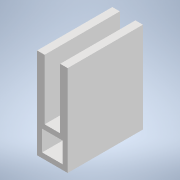
# Autodesk Inventor part: fuselage_tail_interface_front
Saved by Autodesk Inventor 2021 (Build 250183000, 183)
## iProperties
Created: 2020-12-06
Part Number: fuselage_tail_interface_front
Material: Generic
Document SubType Name: Modeling
Designer: victo
Density: 1 g/cm^3
Appearance: Default
Mass: 0.846 g
Surface Area: 14.448 cm^2
Volume: 0.846 cm^3
Author: victo
Autodesk Inventor part; units mm, degrees
ref_plane "YZ Plane" through (0, 0, 0) normal (1, 0, 0) x (0, 1, 0)
ref_plane "XZ Plane" through (0, 0, 0) normal (0, 1, 0) x (-1, 0, 0)
ref_plane "XY Plane" through (0, 0, 0) normal (0, 0, 1) x (1, 0, 0)
sketch "Sketch1" plane through (0, 0, 0) normal (0, 0, 1) x (1, 0, 0)
  line L0 (-3.05, 3.05) -> (3.05, 3.05)
  line L1 (3.05, 3.05) -> (3.05, -3.05)
  line L2 (3.05, -3.05) -> (-3.05, -3.05)
  line L3 (-3.05, -3.05) -> (-3.05, 3.05)
  line L4 (-3.05, 3.05) -> (3.05, -3.05) construction
  line L5 (3.05, 3.05) -> (-3.05, -3.05) construction
  line L6 (-2.05, 2.05) -> (2.05, 2.05)
  line L7 (2.05, 2.05) -> (2.05, -2.05)
  line L8 (2.05, -2.05) -> (-2.05, -2.05)
  line L9 (-2.05, -2.05) -> (-2.05, 2.05)
  line L10 (-2.05, 2.05) -> (2.05, -2.05) construction
  line L11 (2.05, 2.05) -> (-2.05, -2.05) construction
  line L12 (-3.05, 3.05) -> (-1.55, 3.05)
  line L13 (-1.55, 3.05) -> (-1.55, 15.05)
  line L14 (-1.55, 15.05) -> (-3.05, 15.05)
  line L15 (-3.05, 15.05) -> (-3.05, 3.05)
  line L16 (3.05, 3.05) -> (1.55, 3.05)
  line L17 (1.55, 3.05) -> (1.55, 15.05)
  line L18 (1.55, 15.05) -> (3.05, 15.05)
  line L19 (3.05, 15.05) -> (3.05, 3.05)
  point P0 (0, 0)
  point P1 (1.55, 3.05)
  point P2 (-1.55, 3.05)
  dimension "d0" = 6.1
  dimension "d1" = 6.1
  dimension "d2" = 4.1
  dimension "d3" = 4.1
  dimension "d4" = 12
  dimension "d5" = 12
  dimension "d6" = 1.5
  dimension "d7" = 1.5
  constraints: 40 end point, 8 parallel, 4 horizontal, 4 midpoint, 4 perpendicular, 2 point on line
  measures "d0" distance of L0.end L1.end
  measures "d1" distance of L1.end L2.end
  measures "d2" distance of L6.end L7.end
  measures "d3" distance of L6.start L6.end
  measures "d4" distance of L18.end L16.start
  measures "d5" distance of L14.end L0.start
  measures "d6" distance of L13.end L14.end
  measures "d7" distance of L17.end L18.end
extrude "Extrusion1" add sketch "Sketch1" along normal blind 15
body "Solid1"
